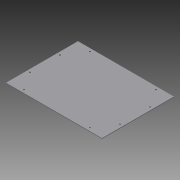
# Autodesk Inventor part: 000103
Saved by Autodesk Inventor 2015 (Build 190159000, 159)
## iProperties
Created: 2015-05-11
Part Number: 000103
Material: Generic
Document SubType Name: Modeling
Designer: Wesley
Density: 1 g/cm^3
Appearance: Default
Author: Wesley
Autodesk Inventor part; units mm, degrees
ref_plane "YZ Plane" through (0, 0, 0) normal (1, 0, 0) x (0, 1, 0)
ref_plane "XZ Plane" through (0, 0, 0) normal (0, 1, 0) x (-1, 0, 0)
ref_plane "XY Plane" through (0, 0, 0) normal (0, 0, 1) x (1, 0, 0)
sketch "Sketch1" plane through (0, 0, 0) normal (0, 1, 0) x (-1, 0, 0)
  line L0 (0, 0) -> (203.2, 0)
  line L1 (203.2, 0) -> (203.2, -152.4)
  line L2 (203.2, -152.4) -> (0, -152.4)
  line L3 (0, -152.4) -> (0, 0)
  dimension "d0" = 203.2
  dimension "d1" = 152.4
  constraints: 8 end point, 2 parallel, 1 horizontal, 1 perpendicular
  measures "d0" distance of L0.start L0.end
  measures "d1" distance of L2.end L0.start
extrude "Extrusion1" add sketch "Sketch1" along normal blind 1.27
sketch "Sketch3" plane through (0, 1.27, 0) normal (0, 1, 0) x (1, 0, 0)
  circle A0 centre (-171.45, 6.35) radius 1.5875
  circle A1 centre (-196.8524, 44.45) radius 1.5875
  circle A2 centre (-31.75, 6.35) radius 1.5875
  circle A3 centre (-6.35, 44.45) radius 1.5875
  circle A4 centre (-6.35, 107.95) radius 1.5875
  circle A5 centre (-31.75, 146.05) radius 1.5875
  circle A6 centre (-171.45, 146.05) radius 1.5875
  circle A7 centre (-196.85, 107.95) radius 1.5875
  line L0 (-203.2, 152.4) -> (-203.2, 0) projected
  line L1 (0, 152.4) -> (-203.2, 152.4) projected
  line L2 (0, 0) -> (0, 152.4) projected
  line L3 (-203.2, 0) -> (0, 0) projected
  dimension "d36" = 3.175
  dimension "d37" = 3.175
  dimension "d38" = 3.175
  dimension "d39" = 3.175
  dimension "d40" = 3.175
  dimension "d41" = 3.175
  dimension "d42" = 3.175
  dimension "d43" = 3.175
  dimension "d45" = 6.35
  dimension "d46" = 44.45
  dimension "d47" = 6.35
  dimension "d48" = 31.75
  dimension "d49" = 31.75
  dimension "d50" = 6.35
  dimension "d51" = 44.45
  dimension "d52" = 6.35
  dimension "d53" = 44.45
  dimension "d54" = 6.35
  dimension "d55" = 31.75
  dimension "d56" = 6.35
  dimension "d57" = 31.75
  dimension "d58" = 6.3476
  dimension "d59" = 44.45
  dimension "d62" = 203.2
  dimension "d63" = 152.4
  constraints: 8 centre point, 8 coincident, 1 horizontal alignment
  measures "d36" diameter of A0
  measures "d37" diameter of A1
  measures "d38" diameter of A2
  measures "d39" diameter of A3
  measures "d40" diameter of A4
  measures "d41" diameter of A5
  measures "d42" diameter of A6
  measures "d43" diameter of A7
  measures "d45" distance from line of L0 A7.centre
  measures "d46" distance from line of L1 A7.centre
  measures "d47" distance from line of L1 A6.centre
  measures "d48" distance from line of L0 A6.centre
  measures "d49" distance from line of L2 point (-31.75, 146.05)
  measures "d50" distance from line of L2 point (-6.35, 107.95)
  measures "d51" distance from line of L1 point (-6.35, 107.95)
  measures "d52" distance from line of L2 point (-6.35, 44.45)
  measures "d53" distance from line of L3 point (-6.35, 44.45)
  measures "d54" distance from line of L3 point (-31.75, 6.35)
  measures "d55" distance from line of L2 point (-31.75, 6.35)
  measures "d56" distance from line of L3 point (-171.45, 6.35)
  measures "d57" distance from line of L0 point (-171.45, 6.35)
  measures "d58" distance from line of L0 point (-196.852, 44.45)
  measures "d59" distance from line of L3 point (-196.852, 44.45)
  measures "d62" distance of L0.end L2.start
  measures "d63" distance of L0.start L0.end
extrude "Extrusion2" cut sketch "Sketch3" against normal blind 25.4 contours A0 | A1 | A2 | A3 | A4 | A5 | A6 | A7
body "Solid1"
